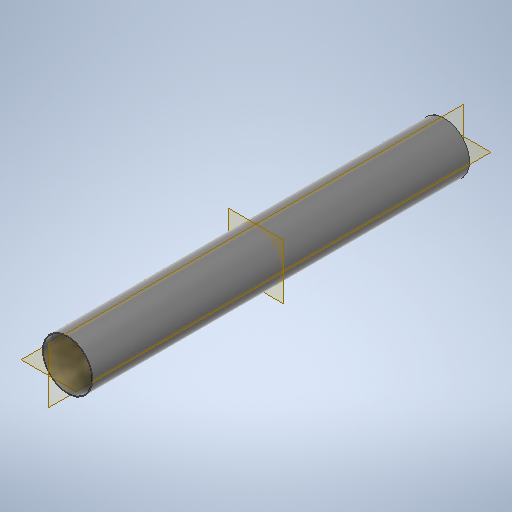
# Autodesk Inventor part: Tubo_0001
Saved by Autodesk Inventor 2025.2 (Build 292293000, 293)
## iProperties
Created: 2025-03-28
Part Number: Tubo_0001
Material: Generic
Document SubType Name: Modeling
Designer: ishad
Density: 1 g/cm^3
Appearance: Default
Author: ishad
Autodesk Inventor part; units mm, degrees
sketch "Sketch1" plane through (0, 0, 0) normal (0, 0, 1) x (1, 0, 0)
  circle A0 centre (0, 0) radius 50
  circle A1 centre (0, 0) radius 48.5
  dimension "d0" = 100
  dimension "d1" = 97
  constraints: 2 centre point, 2 coincident
  measures "d0" diameter of A0
  measures "d1" diameter of A1
extrude "Extrusion1" add sketch "Sketch1" along normal mid plane 750
body "Solid1"
